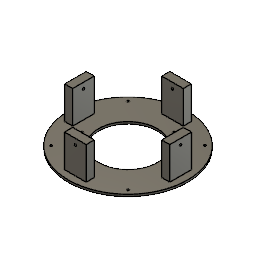
_top_3D Joint.c7dbc639-92e2-42d0-a810-be37d3c962a2 (Autodesk Fusion 360 design; units mm, degrees)
Autodesk Fusion 360 part; units mm, degrees
sketch "Sketch1" plane through (0, 0, 0) normal (0, 1, 0) x (1, 0, 0)
  circle A0 centre (0, 0) radius 27
  circle A1 centre (0, 0) radius 55
  line L0 (10, -41) -> (-10, -41)
  line L1 (-10, -41) -> (-10, -48.5)
  line L2 (-10, -48.5) -> (10, -48.5)
  line L3 (10, -48.5) -> (10, -41)
  line L4 (10, -41) -> (-10, -48.5) construction
  line L5 (-10, -41) -> (10, -48.5) construction
  line L6 (41, 10) -> (48.5, -10) construction
  line L7 (41, 10) -> (41, -10)
  line L8 (48.5, -10) -> (48.5, 10)
  line L9 (48.5, 10) -> (41, 10)
  line L10 (41, -10) -> (48.5, 10) construction
  line L11 (41, -10) -> (48.5, -10)
  line L12 (-10, 41) -> (10, 48.5) construction
  line L13 (-10, 41) -> (10, 41)
  line L14 (10, 48.5) -> (-10, 48.5)
  line L15 (-10, 48.5) -> (-10, 41)
  line L16 (10, 41) -> (-10, 48.5) construction
  line L17 (10, 41) -> (10, 48.5)
  line L18 (-41, -10) -> (-48.5, 10) construction
  line L19 (-41, -10) -> (-41, 10)
  line L20 (-48.5, 10) -> (-48.5, -10)
  line L21 (-48.5, -10) -> (-41, -10)
  line L22 (-41, 10) -> (-48.5, -10) construction
  line L23 (-41, 10) -> (-48.5, 10)
  line L24 (0, 0) -> (0, -44.75)
  line L25 (0, 0) -> (27, 0)
  point P0 (0, -44.75)
  point P1 (44.75, 0)
  point P2 (0, 44.75)
  point P3 (-44.75, 0)
  dimension "d1" = 54
  dimension "d2" = 110
  dimension "d7" = 7.5
  dimension "d8" = 20
  dimension "d9" = 41
  dimension "d11" = 360
  measures "d1" diameter of A0
  measures "d2" diameter of A1
  measures "d7" distance of L0.end L1.end
  measures "d8" distance of L1.end L2.end
  measures "d9" distance of A0.centre L0
extrude "Extrude3" add sketch "Sketch1" along normal blind 2 contours A1 | L0 L1 L2 L3 | L7 L8 L9 L11 | L13 L14 L15 L17 | L19 L20 L21 L23
extrude "Extrude5" add sketch "Sketch1" along normal blind 32 contours L0 L1 L2 L3 | L7 L8 L9 L11 | L13 L14 L15 L17 | L19 L20 L21 L23
sketch "Sketch6" plane through (0, 2, 0) normal (0, 1, 0) x (-1, 0, 0)
  line L0 (-10, 48.5) -> (10, 48.5)
  line L1 (10, 48.5) -> (10, 41)
  line L2 (10, 41) -> (-10, 41)
  line L3 (-10, 41) -> (-10, 48.5)
  line L4 (41, -10) -> (41, 10)
  line L5 (41, 10) -> (48.5, 10)
  line L6 (48.5, 10) -> (48.5, -10)
  line L7 (48.5, -10) -> (41, -10)
  line L8 (-41, 10) -> (-41, -10)
  line L9 (-41, -10) -> (-48.5, -10)
  line L10 (-48.5, -10) -> (-48.5, 10)
  line L11 (-48.5, 10) -> (-41, 10)
  line L12 (-10, -41) -> (10, -41)
  line L13 (10, -41) -> (10, -48.5)
  line L14 (10, -48.5) -> (-10, -48.5)
  line L15 (-10, -48.5) -> (-10, -41)
  circle A0 centre (0, 0) radius 27
  circle A1 centre (0, 0) radius 55
  line L16 (29.6985, 15.5563) -> (26.8701, 12.7279)
  line L17 (12.7279, 26.8701) -> (15.5563, 29.6985)
  line L18 (18.1297, 22.7228) -> (20.9915, 22.7228) construction
  line L19 (15.3614, 25.1762) -> (18.4198, 25.1762) construction
  line L20 (17.8019, 25.9553) -> (17.4822, 25.9553) construction
  line L21 (29.6985, 15.5563) -> (26.8701, 12.7279)
  line L22 (26.8701, 12.7279) -> (22.6274, 16.9706)
  line L23 (22.6274, 16.9706) -> (25.4558, 19.799)
  line L24 (25.4558, 19.799) -> (29.6985, 15.5563)
  line L25 (15.5563, 29.6985) -> (12.7279, 26.8701)
  line L26 (12.7279, 26.8701) -> (16.9706, 22.6274)
  line L27 (16.9706, 22.6274) -> (19.799, 25.4558)
  line L28 (19.799, 25.4558) -> (15.5563, 29.6985)
  line L29 (22.6274, 16.9706) -> (16.9706, 22.6274)
  line L30 (0, 0) -> (27, 0)
  line L31 (0, 0) -> (19.799, 19.799)
  line L32 (-15.3614, -25.1762) -> (-18.4198, -25.1762) construction
  line L33 (-22.6274, -16.9706) -> (-25.4558, -19.799)
  line L34 (-12.7279, -26.8701) -> (-15.5563, -29.6985)
  line L35 (-26.8701, -12.7279) -> (-22.6274, -16.9706)
  line L36 (-12.7279, -26.8701) -> (-16.9706, -22.6274)
  line L37 (-25.4558, -19.799) -> (-29.6985, -15.5563)
  line L38 (-29.6985, -15.5563) -> (-26.8701, -12.7279)
  line L39 (-18.1297, -22.7228) -> (-20.9915, -22.7228) construction
  line L40 (-29.6985, -15.5563) -> (-26.8701, -12.7279)
  line L41 (-19.799, -25.4558) -> (-15.5563, -29.6985)
  line L42 (-16.9706, -22.6274) -> (-19.799, -25.4558)
  line L43 (-22.6274, -16.9706) -> (-16.9706, -22.6274)
  line L44 (-15.5563, -29.6985) -> (-12.7279, -26.8701)
  line L45 (-17.8019, -25.9553) -> (-17.4822, -25.9553) construction
  circle A2 centre (35.3553, -35.3553) radius 1
  line L46 (35.3553, -35.3553) -> (0, 0)
  circle A3 centre (35.3553, 35.3553) radius 1
  circle A4 centre (-35.3553, 35.3553) radius 1
  circle A5 centre (-35.3553, -35.3553) radius 1
  circle A6 centre (31.8198, 10.6066) radius 1
  line L47 (28.2843, 14.1421) -> (31.8198, 10.6066)
  line L48 (19.799, 19.799) -> (22.225, 22.225)
  circle A7 centre (10.6066, 31.8198) radius 1
  circle A8 centre (-31.8198, -10.6066) radius 1
  circle A9 centre (-10.6066, -31.8198) radius 1
  point P0 (19.799, 19.799)
  point P1 (-19.799, -19.799)
  point P2 (-19.799, -19.799)
  dimension "d37" = 4
  dimension "d38" = 20
  dimension "d43" = 6
  dimension "d44" = 6
  dimension "d45" = 4
  dimension "d46" = 45
  dimension "d48" = 360
  dimension "d61" = 2
  dimension "d62" = 45
  dimension "d63" = 50
  dimension "d65" = 360
  dimension "d68" = 2
  dimension "d69" = 5
  dimension "d71" = 360
  dimension "d74" = 16
  dimension "d75" = 28
  measures "d37" distance of L16.start L16.end
  measures "d38" distance of L16.start L17.end
  measures "d43" distance of L16.start L23.end
  measures "d44" distance of L17.end L27.end
  measures "d45" distance of L26 L28
  measures "d46" angle of L30 L31
  measures "d61" diameter of A2
  measures "d62" angle of L30 L46
  measures "d63" distance of A0.centre A2.centre
  measures "d68" diameter of A6
  measures "d69" distance of L21 A6.centre
  measures "d75" distance of A0.centre P0
extrude "Extrude12" cut sketch "Sketch6" against normal blind 30 contours A6 | A7 | A8 | A9
extrude "Extrude11" cut sketch "Sketch6" against normal blind 10 contours A2 | A3 | A4 | A5
sketch "Sketch8" plane through (0, 0, 48.5) normal (0, 0, 1) x (1, 0, 0)
  line L0 (-10, 2) -> (10, 2)
  line L1 (10, 2) -> (10, 32)
  line L2 (10, 32) -> (-10, 32)
  line L3 (-10, 32) -> (-10, 2)
  circle A0 centre (0, 26.7) radius 1
  dimension "d51" = 2
  dimension "d52" = 10
  dimension "d53" = 24.7
  measures "d51" diameter of A0
  measures "d52" distance of L1 A0.centre
  measures "d53" distance of L0 A0.centre
extrude "Extrude9" cut sketch "Sketch8" against normal blind 100 contours A0
sketch "Sketch9" plane through (48.5, 0, 0) normal (1, 0, 0) x (0, 0, -1)
  line L0 (-10, 2) -> (10, 2)
  line L1 (10, 2) -> (10, 32)
  line L2 (10, 32) -> (-10, 32)
  line L3 (-10, 32) -> (-10, 2)
  circle A0 centre (0, 26.7) radius 1
  dimension "d56" = 2
  dimension "d57" = 10
  dimension "d58" = 24.7
  measures "d56" diameter of A0
  measures "d57" distance of L1 A0.centre
  measures "d58" distance of L0 A0.centre
extrude "Extrude10" cut sketch "Sketch9" against normal blind 100 contours A0
sketch "Sketch10" plane through (0, 2, 0) normal (0, 1, 0) x (-1, 0, 0)
  circle A0 centre (35.3553, 35.3553) radius 1
  circle A1 centre (-35.3553, 35.3553) radius 1
  circle A2 centre (35.3553, -35.3553) radius 1
  circle A3 centre (-35.3553, -35.3553) radius 1
  circle A4 centre (-31.8198, -10.6066) radius 1
  circle A5 centre (31.8198, 10.6066) radius 1
  circle A6 centre (-10.6066, -31.8198) radius 1
  circle A7 centre (10.6066, 31.8198) radius 1
  line L0 (-10, 48.5) -> (10, 48.5)
  line L1 (10, 48.5) -> (10, 41)
  line L2 (10, 41) -> (-10, 41)
  line L3 (-10, 41) -> (-10, 48.5)
  line L4 (41, -10) -> (41, 10)
  line L5 (41, 10) -> (48.5, 10)
  line L6 (48.5, 10) -> (48.5, -10)
  line L7 (48.5, -10) -> (41, -10)
  line L8 (-41, 10) -> (-41, -10)
  line L9 (-41, -10) -> (-48.5, -10)
  line L10 (-48.5, -10) -> (-48.5, 10)
  line L11 (-48.5, 10) -> (-41, 10)
  line L12 (-10, -41) -> (10, -41)
  line L13 (10, -41) -> (10, -48.5)
  line L14 (10, -48.5) -> (-10, -48.5)
  line L15 (-10, -48.5) -> (-10, -41)
  circle A8 centre (0, 0) radius 27
  circle A9 centre (0, 0) radius 55
